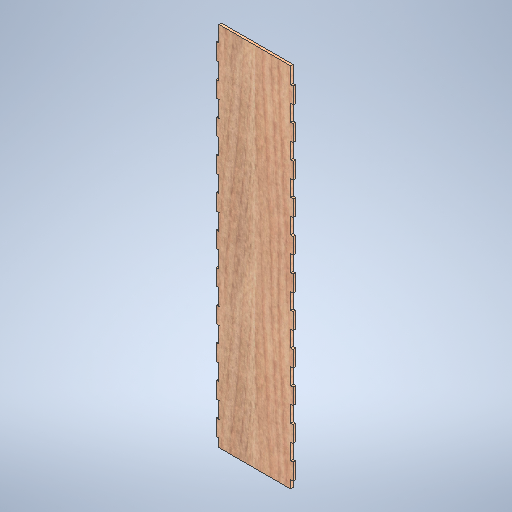
# Autodesk Inventor part: Part1 box
Saved by Autodesk Inventor 2025.3 (Build 293356000, 356)
## iProperties
Created: 2026-04-05
Part Number: Part1 box
Material: Wood (Birch)
Document SubType Name: Modeling
Designer: logien
Density: 0.55 g/cm^3
Appearance: Birch - Natural Polished
Author: logien
Autodesk Inventor part; units mm, degrees
ref_plane "YZ Plane" through (0, 0, 0) normal (1, 0, 0) x (0, 1, 0)
ref_plane "XZ Plane" through (0, 0, 0) normal (0, 1, 0) x (-1, 0, 0)
ref_plane "XY Plane" through (0, 0, 0) normal (0, 0, 1) x (1, 0, 0)
sketch "Sketch1" plane through (0, 0, 0) normal (0, 0, 1) x (1, 0, 0)
  line L0 (0, 0) -> (88, 0)
  line L1 (88, 10) -> (91, 10)
  line L2 (91, 10) -> (91, 30)
  line L3 (91, 30) -> (88, 30)
  line L4 (91, 50) -> (91, 70)
  line L5 (91, 70) -> (88, 70)
  line L6 (88, 70) -> (88, 90)
  line L7 (88, 90) -> (91, 90)
  line L8 (91, 90) -> (91, 110)
  line L9 (91, 110) -> (88, 110)
  line L10 (88, 110) -> (88, 130)
  line L11 (88, 130) -> (91, 130)
  line L12 (91, 130) -> (91, 150)
  line L13 (91, 150) -> (88, 150)
  line L14 (88, 150) -> (88, 170)
  line L15 (88, 170) -> (91, 170)
  line L16 (91, 170) -> (91, 190)
  line L17 (91, 190) -> (88, 190)
  line L18 (88, 190) -> (88, 210)
  line L19 (88, 210) -> (91, 210)
  line L20 (91, 210) -> (91, 230)
  line L21 (91, 230) -> (88, 230)
  line L22 (88, 230) -> (88, 250)
  line L23 (88, 250) -> (91, 250)
  line L24 (91, 250) -> (91, 270)
  line L25 (91, 270) -> (88, 270)
  line L26 (88, 270) -> (88, 290)
  line L27 (88, 290) -> (91, 290)
  line L28 (91, 290) -> (91, 310)
  line L29 (91, 310) -> (88, 310)
  line L30 (88, 310) -> (88, 330)
  line L31 (88, 330) -> (91, 330)
  line L32 (91, 330) -> (91, 350)
  line L33 (91, 350) -> (88, 350)
  line L34 (88, 350) -> (88, 370)
  line L35 (88, 370) -> (91, 370)
  line L36 (91, 370) -> (91, 390)
  line L37 (91, 390) -> (88, 390)
  line L38 (88, 390) -> (88, 410)
  line L39 (88, 410) -> (91, 410)
  line L40 (91, 410) -> (91, 430)
  line L41 (91, 430) -> (88, 430)
  line L42 (44, 0) -> (44, 110) construction
  line L43 (0, 10) -> (-3, 10)
  line L44 (-3, 10) -> (-3, 30)
  line L45 (-3, 30) -> (0, 30)
  line L46 (-3, 50) -> (-3, 70)
  line L47 (-3, 70) -> (0, 70)
  line L48 (0, 70) -> (0, 90)
  line L49 (0, 90) -> (-3, 90)
  line L50 (-3, 90) -> (-3, 110)
  line L51 (-3, 110) -> (0, 110)
  line L52 (0, 110) -> (0, 130)
  line L53 (0, 130) -> (-3, 130)
  line L54 (-3, 130) -> (-3, 150)
  line L55 (-3, 150) -> (0, 150)
  line L56 (0, 150) -> (0, 170)
  line L57 (0, 170) -> (-3, 170)
  line L58 (-3, 170) -> (-3, 190)
  line L59 (-3, 190) -> (0, 190)
  line L60 (0, 190) -> (0, 210)
  line L61 (0, 210) -> (-3, 210)
  line L62 (-3, 210) -> (-3, 230)
  line L63 (-3, 230) -> (0, 230)
  line L64 (0, 230) -> (0, 250)
  line L65 (0, 250) -> (-3, 250)
  line L66 (-3, 250) -> (-3, 270)
  line L67 (-3, 270) -> (0, 270)
  line L68 (0, 270) -> (0, 290)
  line L69 (0, 290) -> (-3, 290)
  line L70 (-3, 290) -> (-3, 310)
  line L71 (-3, 310) -> (0, 310)
  line L72 (0, 310) -> (0, 330)
  line L73 (0, 330) -> (-3, 330)
  line L74 (-3, 330) -> (-3, 350)
  line L75 (-3, 350) -> (0, 350)
  line L76 (0, 350) -> (0, 370)
  line L77 (0, 370) -> (-3, 370)
  line L78 (-3, 370) -> (-3, 390)
  line L79 (-3, 390) -> (0, 390)
  line L80 (0, 390) -> (0, 410)
  line L81 (0, 410) -> (-3, 410)
  line L82 (-3, 410) -> (-3, 430)
  line L83 (-3, 430) -> (0, 430)
  line L84 (0, 430) -> (0, 450)
  line L85 (0, 450) -> (88, 450)
  line L86 (88, 450) -> (88, 430)
  line L87 (-3, 0) -> (0, 0)
  line L88 (88, 0) -> (91, 0)
  line L89 (-3, 50) -> (0, 50)
  line L90 (0, 50) -> (0, 30)
  line L91 (91, 50) -> (88, 50)
  line L92 (88, 50) -> (88, 30)
  line L93 (88, 10) -> (88, 0)
  line L94 (0, 10) -> (0, 0)
  dimension "d0" = 88
  dimension "d1" = 10
  dimension "d2" = 3
  dimension "d3" = 20
  dimension "d5" = 20
  dimension "d6" = 20
  dimension "d7" = 20
  dimension "d8" = 20
  dimension "d9" = 20
  dimension "d10" = 3
  dimension "d11" = 20
  dimension "d12" = 20
  dimension "d13" = 20
  dimension "d14" = 3
  dimension "d15" = 20
  dimension "d16" = 3
  dimension "d17" = 20
  dimension "d18" = 20
  dimension "d19" = 20
  dimension "d20" = 3
  dimension "d21" = 20
  dimension "d22" = 20
  dimension "d23" = 20
  dimension "d24" = 20
  dimension "d25" = 20
  dimension "d26" = 20
  dimension "d27" = 20
  dimension "d28" = 20
  dimension "d43" = 0
  dimension "d44" = 0
  dimension "d45" = 0
  dimension "d47" = 3
  dimension "d51" = 20
  dimension "d52" = 320
  constraints: 190 end point, 43 point on line, 43 symmetric about line, 25 perpendicular, 8 horizontal, 3 vertical, 1 collinear, 1 midpoint, 1 parallel
  measures "d0" distance of L0.start L0.end
  measures "d1" distance of L0.end L1.start
  measures "d2" distance of L1.start L1.end
  measures "d3" distance of L1.end L2.end
  measures "d5" distance of L3.end L91.end
  measures "d6" distance of L4.start L4.end
  measures "d7" distance of L5.end L6.end
  measures "d8" distance of L7.end L8.end
  measures "d9" distance of L9.end L10.end
  measures "d10" distance of L10.end L11.end
  measures "d11" distance of L11.end L12.end
  measures "d12" distance of L13.end L14.end
  measures "d13" distance of L15.end L16.end
  measures "d14" distance of L16.end L17.end
  measures "d15" distance of L17.end L18.end
  measures "d16" distance of L18.end L19.end
  measures "d17" distance of L19.end L20.end
  measures "d18" distance of L21.end L22.end
  measures "d19" distance of L23.end L24.end
  measures "d20" distance of L24.end L25.end
  measures "d21" distance of L25.end L26.end
  measures "d22" distance of L27.end L28.end
  measures "d23" distance of L29.end L30.end
  measures "d24" distance of L31.end L32.end
  measures "d25" distance of L33.end L34.end
  measures "d26" distance of L35.end L36.end
  measures "d27" distance of L37.end L38.end
  measures "d28" distance of L39.end L40.end
  measures "d43" distance between parallel lines of L36 L32
  measures "d44" distance between parallel lines of L36 L16
  measures "d45" distance between parallel lines of L36 L12
  measures "d47" distance between parallel lines of L38 L36
  measures "d51" distance of L83.end L84.end
  measures "d52" distance from line of L42.end L41
extrude "Extrusion1" add sketch "Sketch1" along normal blind 3
body "Solid1"
